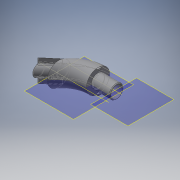
# Autodesk Inventor part: goulot
Saved by Autodesk Inventor 2016 (Build 200138000, 138)
## iProperties
Created: 2016-05-09
Part Number: goulot
Material: Générique
Document SubType Name: Modeling
Designer: Ropert
Density: 1 g/cm^3
Appearance: Par défaut
Author: Ropert
Autodesk Inventor part; units mm, degrees
ref_plane "YZ Plane" through (0, 0, 0) normal (1, 0, 0) x (0, 1, 0)
ref_plane "XZ Plane" through (0, 0, 0) normal (0, 1, 0) x (-1, 0, 0)
ref_plane "XY Plane" through (0, 0, 0) normal (0, 0, 1) x (1, 0, 0)
sketch "Esquisse1" plane through (0, 0, 0) normal (0, 0, 1) x (1, 0, 0)
  arc A0 (30, 15.628789) -> (0, 0) centre (29.157317, -19.361065) ccw
  dimension "d2" = 35
  constraints: 2 point on circle, 1 centre point
  measures "d2" radius of A0
sketch "Esquisse2" plane through (0, 0, 0) normal (1, 0, 0) x (0, 1, 0)
  circle A0 centre (25, 0) radius 13.5
  point P0 (0, 0)
  dimension "d4" = 27
  constraints: 1 centre point
  measures "d4" diameter of A0
sweep "Balayage1" add profiles "Esquisse2" path "Esquisse1" keep normal constant yes
sketch "Esquisse3" plane through (30, 40.628789, 0) normal (1, 0, 0) x (0, 0, -1)
  circle A0 centre (0, 0) radius 8
  circle A1 centre (0, 0) radius 7
  point P0 (0, -40.628789)
  dimension "d7" = 16
  dimension "d8" = 14
  constraints: 2 centre point, 1 coincident
  measures "d7" diameter of A0
  measures "d8" diameter of A1
extrude "Extrusion1" add sketch "Esquisse3" along normal blind 22
ref_plane "Plan de construction1" through (30, 40.628789, 0) normal (0, 0, -1) x (1, 0, 0)
sketch "Esquisse4" plane through (30, 40.628789, 0) normal (1, 0, 0) x (0, 0, -1)
  line L0 (0, -2.128789) -> (0, 13.5)
  circle A0 centre (0, 0.033445) radius 7.00008
  point P0 (0, -40.628789)
  constraints: 1 centre point, 1 point on line
sketch "Esquisse6" plane through (30, 40.628789, 0) normal (0, 0, -1) x (1, 0, 0)
  arc A0 (-30.3, 17.212781) -> (1.67582, 6.176207) centre (-4.314624, 40.659748) ccw
  dimension "d24" = 35
  constraints: 2 point on circle, 1 centre point
  measures "d24" radius of A0
sweep "Balayage2" cut profiles "Esquisse4" path "Esquisse6" keep normal constant yes
fillet "Congé1" radius 1 1 edges at (52, 40.6288, 8)
sketch "Esquisse8" plane through (30, 40.628789, 0) normal (1, 0, 0) x (0, 0, -1)
  line L0 (13.321125, 2.19035) -> (11.85, 2.19035)
  line L1 (11.85, 2.19035) -> (11.85, 0)
  line L2 (11.85, 0) -> (11.85, -2.19035)
  line L3 (13.321125, -2.19035) -> (11.85, -2.19035)
  arc A0 (13.5, 0) -> (13.321125, 2.19035) centre (0, 0) ccw
  arc A1 (13.321125, -2.19035) -> (13.5, 0) centre (0, 0) ccw
  line L4 (-13.321125, -2.19035) -> (-11.85, -2.19035)
  line L5 (-11.85, -2.19035) -> (-11.85, 0)
  line L6 (-11.85, 0) -> (-11.85, 2.19035)
  line L7 (-13.321125, 2.19035) -> (-11.85, 2.19035)
  arc A2 (-13.5, 0) -> (-13.321125, -2.19035) centre (0, 0) ccw
  arc A3 (-13.321125, 2.19035) -> (-13.5, 0) centre (0, 0) ccw
  point P0 (0, -40.628789)
  point P1 (0, 13.5)
  constraints: 16 end point, 8 point on circle, 4 centre point, 2 perpendicular
extrude "Extrusion3" add sketch "Esquisse8" along normal blind 2
ref_plane "Plan de construction2" through (0, 25, 0) normal (0, 0, -1) x (-1, 0, 0)
sketch "Esquisse10" plane through (0, 25, 0) normal (-1, 0, 0) x (0, 0, 1)
  circle A0 centre (0, 4.698076) radius 7.009215
  point P0 (0, -25)
  constraints: 1 centre point
sketch "Esquisse11" plane through (30, 40.628789, 0) normal (0, 0, -1) x (1, 0, 0)
  line L0 (-30, 10.902592) -> (-45.238276, 23.85616)
  point P0 (-30, 40.628789)
  dimension "d25" = 20
  constraints: 2 end point
  measures "d25" distance of L0.start L0.end
sweep "Balayage3" add profiles "Esquisse10" path "Esquisse11"
sketch "Esquisse12" plane through (30, 40.628789, 0) normal (0, 0, -1) x (1, 0, 0)
  line L0 (-30, 10.902592) -> (-45.238276, 23.85616)
  point P0 (-30, 40.628789)
  dimension "d28" = 20
  constraints: 2 end point
  measures "d28" distance of L0.start L0.end
sketch "Esquisse13" plane through (-15.238276, 16.744508, 0) normal (-1, 0, 0) x (0, 0, 1)
  circle A0 centre (0, 0) radius 6
  point P0 (0, -16.744508)
  dimension "d29" = 12
  constraints: 1 centre point
  measures "d29" diameter of A0
sweep "Balayage4" cut profiles "Esquisse13" path "Esquisse12"
sketch "Esquisse14" plane through (0, 25, 0) normal (-1, 0, 0) x (0, 0, 1)
  line L0 (-7.00008, 4.704422) -> (-12.65379, 4.704422)
  line L1 (12.65379, 4.704422) -> (7.009212, 4.704422)
  line L2 (-6.938425, 3.704422) -> (-12.981805, 3.704422)
  line L3 (12.981805, 3.704422) -> (6.938425, 3.704422)
  arc A0 (-12.65379, 4.704422) -> (-12.981805, 3.704422) centre (0, 0) ccw
  arc A1 (-7.00008, 4.704422) -> (-6.938425, 3.704422) centre (-1.172537, 4.561817) ccw
  arc A2 (6.938425, 3.704422) -> (7.009212, 4.704422) centre (0, 4.698076) ccw
  arc A3 (12.981805, 3.704422) -> (12.65379, 4.704422) centre (0, 0) ccw
  point P0 (0, -25)
  point P1 (-7.00008, 15.412735)
  point P2 (0, 13.5)
  dimension "d32" = 1
  dimension "d33" = 1
  constraints: 8 end point, 8 point on circle, 4 centre point, 2 parallel
  measures "d32" distance between parallel lines of L0 L2
  measures "d33" distance between parallel lines of L1 L3
sketch "Esquisse15" plane through (30, 40.628789, 0) normal (0, 0, -1) x (1, 0, 0)
  line L0 (-30, 10.902592) -> (-45.238276, 23.85616)
  point P0 (-30, 40.628789)
  point P1 (-30, 40.628789)
  dimension "d34" = 20
  constraints: 2 end point
  measures "d34" distance of L0.start L0.end
sweep "Balayage5" add profiles "Esquisse14" path "Esquisse15"
fillet "Congé2" radius 2 1 edges at (-7.6191, 23.2276, 7.0092)
fillet "Congé3" radius 2 1 edges at (-7.6191, 22.2276, 6.9384)
fillet "Congé4" radius 2 1 edges at (-7.6191, 23.2276, -7.0092)
sketch "Esquisse16" plane through (0, 25, 0) normal (-1, 0, 0) x (0, 0, 1)
  arc A0 (-6.938425, 3.704422) -> (6.563363, 2.238125) centre (0, 4.698076) ccw
  line L0 (0, 29.138935) -> (0, 13.5)
  circle A1 centre (0, -7.311139) radius 1.5
  point P0 (0, -25)
  point P1 (0, 29.128789)
  dimension "d41" = 3
  constraints: 1 centre point
  measures "d41" diameter of A1
extrude "Extrusion4" cut sketch "Esquisse16" against normal blind 2.5
